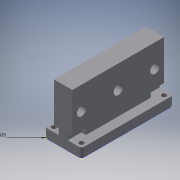
# Autodesk Inventor part: Far Gantry Bracket
Saved by Autodesk Inventor 2016 (Build 200138000, 138)
## iProperties
Created: 2016-04-12
Part Number: Far Gantry Bracket
Material: Generic
Document SubType Name: Modeling
Designer: rubenjm
Density: 1 g/cm^3
Appearance: Default
Author: rubenjm
Autodesk Inventor part; units mm, degrees
ref_plane "YZ Plane" through (0, 0, 0) normal (1, 0, 0) x (0, 1, 0)
ref_plane "XZ Plane" through (0, 0, 0) normal (0, 1, 0) x (-1, 0, 0)
ref_plane "XY Plane" through (0, 0, 0) normal (0, 0, 1) x (1, 0, 0)
sketch "Sketch1" plane through (0, 0, 0) normal (0, 1, 0) x (-1, 0, 0)
  line L0 (3.175, 0) -> (47.625, 0)
  line L1 (50.8, -3.175) -> (50.8, -123.825)
  line L2 (47.625, -127) -> (3.175, -127)
  line L3 (0, -123.825) -> (0, -3.175)
  arc A0 (50.8, -3.175) -> (47.625, 0) centre (47.625, -3.175) ccw
  arc A1 (3.175, 0) -> (0, -3.175) centre (3.175, -3.175) ccw
  arc A2 (0, -123.825) -> (3.175, -127) centre (3.175, -123.825) ccw
  arc A3 (47.625, -127) -> (50.8, -123.825) centre (47.625, -123.825) ccw
  point P0 (0, 0)
  point P1 (50.8, -127)
  point P2 (50.8, 0)
  point P3 (0, -127)
  dimension "d0" = 50.8
  dimension "d1" = 127
  dimension "d4" = 3.175
  constraints: 8 end point, 8 point on circle, 8 point on line, 8 tangent, 4 centre point, 3 equal radius, 2 parallel, 1 horizontal, 1 perpendicular
  measures "d0" distance of point (50.8, -127) point (0, -127)
  measures "d1" distance of point (50.8, 0) point (50.8, -127)
  measures "d4" radius of A0
extrude "Extrusion1" add sketch "Sketch1" along normal blind 12.7
sketch "Sketch2" plane through (0, 12.7, 0) normal (0, 1, 0) x (1, 0, 0)
  line L0 (0, 0) -> (-6.35, 0) construction
  line L1 (-6.35, 0) -> (-6.35, 6.35) construction
  line L2 (-6.35, 6.35) -> (0, 6.35) construction
  line L3 (0, 6.35) -> (0, 0) construction
  circle A0 centre (-6.35, 6.35) radius 3.175
  line L4 (0, 3.175) -> (0, 123.825) construction
  line L5 (0, 63.5) -> (-50.8802, 63.5) construction
  line L6 (-50.8802, 63.5) -> (-25.4, 127) construction
  line L7 (-3.175, 127) -> (-47.625, 127) construction
  line L8 (-25.4, 127) -> (-25.4, 0) construction
  line L9 (-47.625, 0) -> (-3.175, 0) construction
  circle A1 centre (-6.35, 120.65) radius 3.175
  circle A2 centre (-44.45, 6.35) radius 3.175
  circle A3 centre (-44.45, 120.65) radius 3.175
  dimension "d5" = 6.35
  dimension "d6" = 6.35
  dimension "d7" = 6.35
  constraints: 14 end point, 4 centre point, 3 midpoint, 3 symmetric about line, 2 horizontal, 2 parallel, 1 coincident, 1 perpendicular, 3 other
  measures "d5" distance of L1.end L2.end
  measures "d6" distance of L0.end L1.end
  measures "d7" diameter of A0
extrude "Extrusion2" cut sketch "Sketch2" against normal through all
sketch "Sketch3" plane through (0, 12.7, 0) normal (0, 1, 0) x (1, 0, 0)
  line L0 (0, 0) -> (-12.7, 0) construction
  line L1 (0, 0) -> (12.7, 0) construction
  line L2 (-47.625, 0) -> (-3.175, 0) construction
  line L3 (-25.4, 0) -> (-25.4, 127) construction
  line L4 (-3.175, 127) -> (-47.625, 127) construction
  line L5 (-50.8, 0) -> (-38.1, 0) construction
  line L6 (-38.1, 0) -> (-12.7, 0)
  line L7 (-12.7, 0) -> (-12.7, 127)
  line L8 (-12.7, 127) -> (-38.1, 127)
  line L9 (-38.1, 127) -> (-38.1, 0)
  dimension "d14" = 12.7
  dimension "d15" = 180
  dimension "d36" = 25.4
  constraints: 16 end point, 3 horizontal, 2 midpoint, 2 parallel, 2 symmetric about line, 1 collinear, 1 perpendicular, 1 point on line
  measures "d14" distance of L0.start L0.end
  measures "d15" angle of L0 L1
  measures "d36" distance of L6.end L5.end
extrude "Extrusion3" add sketch "Sketch3" along normal blind 63.5
sketch "Sketch5" plane through (-12.7, 12.7, 0) normal (1, 0, 0) x (0, 0, -1)
  line L0 (0, 63.5) -> (127, 63.5) construction
  line L1 (63.5, 63.5) -> (63.5, 0) construction
  line L2 (123.825, 0) -> (3.175, 0) construction
  line L3 (127, 0) -> (127, 63.5) construction
  circle A0 centre (63.5, 31.7498) radius 6.35
  circle A1 centre (12.7, 31.7498) radius 6.35
  circle A2 centre (114.3, 31.7498) radius 6.35
  line L4 (0, 0) -> (0, 63.5) construction
  line L5 (0, 31.75) -> (127, 31.75) construction
  point P0 (0, -12.7)
  dimension "d24" = 12.7
  dimension "d27" = 12.7
  dimension "d37" = 50.8
  dimension "d38" = 50.8
  constraints: 4 end point, 4 midpoint, 3 centre point
  measures "d24" diameter of A0
  measures "d27" diameter of A1
  measures "d37" distance of A0.centre A1.centre
  measures "d38" distance of A2.centre A0.centre
extrude "Extrusion5" cut sketch "Sketch5" against normal blind 12.7
sketch "Sketch6" plane through (0, 12.7, 0) normal (0, 1, 0) x (1, 0, 0)
  line L0 (-12.7, 0) -> (-19.05, 0)
  line L1 (-19.05, 0) -> (-19.05, 19.05)
  line L2 (-19.05, 19.05) -> (-12.7, 19.05)
  line L3 (-12.7, 19.05) -> (-12.7, 0)
  line L4 (-38.1, 127) -> (-38.1, 0) construction
  line L5 (-38.4604, 63.7403) -> (-13.0604, 63.7086) construction
  line L6 (-12.7, 69.85) -> (-12.7, 57.15) construction
  line L7 (-12.541, 127.416) -> (-18.891, 127.4319)
  line L8 (-18.891, 127.4319) -> (-18.9385, 108.3819)
  line L9 (-18.9385, 108.3819) -> (-12.5885, 108.3661)
  line L10 (-12.5885, 108.3661) -> (-12.541, 127.416)
  line L11 (-47.625, 0) -> (-3.175, 0) construction
  line L12 (-25.4, 0) -> (-25.4, 127) construction
  line L13 (-3.175, 127) -> (-47.625, 127) construction
  line L14 (-38.1, 0) -> (-31.75, 0)
  line L15 (-31.75, 0) -> (-31.75, 19.05)
  line L16 (-31.75, 19.05) -> (-38.1, 19.05)
  line L17 (-38.1, 19.05) -> (-38.1, 0)
  line L18 (-38.1, 69.85) -> (-38.1, 57.15) construction
  line L19 (-38.259, 127.416) -> (-31.909, 127.4319)
  line L20 (-31.909, 127.4319) -> (-31.8615, 108.3819)
  line L21 (-31.8615, 108.3819) -> (-38.2115, 108.3661)
  line L22 (-38.2115, 108.3661) -> (-38.259, 127.416)
  line L23 (-47.625, 0) -> (-2.456, 0) construction
  point P0 (0, 0)
  point P1 (-37.7396, 63.7086)
  point P2 (-38.1, 69.85)
  point P3 (-38.1, 57.15)
  dimension "d30" = 6.35
  dimension "d31" = 19.05
  constraints: 38 end point, 15 symmetric about line, 2 midpoint, 2 parallel, 1 horizontal, 1 perpendicular, 1 point on line, 3 other
  measures "d30" distance of L1.end L2.end
  measures "d31" distance of L0.end L1.end
extrude "Extrusion6" cut sketch "Sketch6" along normal blind 8.382
sketch "Sketch7" plane through (0, 0, 0) normal (0, -1, 0) x (1, 0, 0)
  line L0 (-3.175, 0) -> (-47.625, 0) construction
  line L1 (-50.8, -3.175) -> (-50.8, -123.825) construction
  line L2 (-47.625, -127) -> (-3.175, -127) construction
  line L3 (0, -123.825) -> (0, -3.175) construction
  circle A0 centre (-44.45, -6.35) radius 3.175 construction
  circle A1 centre (-44.45, -6.35) radius 3.175 construction
  circle A2 centre (-6.35, -6.35) radius 3.175 construction
  circle A3 centre (-6.35, -6.35) radius 3.175 construction
  circle A4 centre (-44.45, -120.65) radius 3.175 construction
  circle A5 centre (-44.45, -120.65) radius 3.175 construction
  circle A6 centre (-6.35, -120.65) radius 3.175 construction
  arc A7 (-47.625, 0) -> (-50.8, -3.175) centre (-47.625, -3.175) ccw construction
  arc A8 (0, -3.175) -> (-3.175, 0) centre (-3.175, -3.175) ccw construction
  arc A9 (-3.175, -127) -> (0, -123.825) centre (-3.175, -123.825) ccw construction
  arc A10 (-50.8, -123.825) -> (-47.625, -127) centre (-47.625, -123.825) ccw construction
  point P0 (0, 0)
  dimension "d39" = 3.175
  constraints: 8 centre point, 8 end point, 8 point on circle, 8 tangent, 3 coincident, 3 equal radius, 2 parallel, 2 point on line, 1 horizontal, 1 perpendicular
  measures "d39" radius of A7
body "Solid1"
